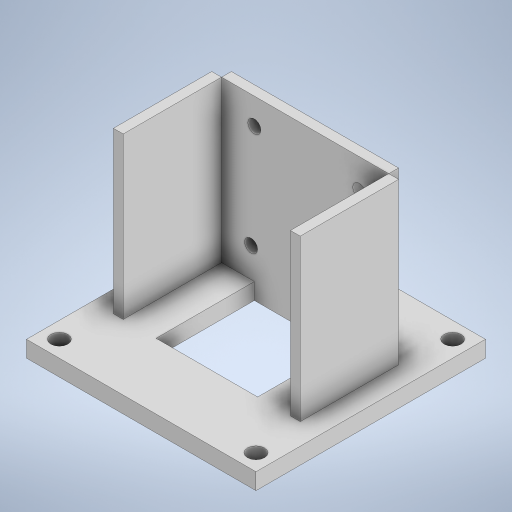
# Autodesk Inventor part: depth_camera_fastening
Saved by Autodesk Inventor 2024 (Build 280153000, 153)
## iProperties
Created: 2024-04-08
Part Number: depth_camera_fastening
Material: Genérico
Document SubType Name: Modeling
Designer: inigo
Density: 1 g/cm^3
Appearance: Valor por defecto
Author: inigo
Autodesk Inventor part; units mm, degrees
ref_plane "YZ Plane" through (0, 0, 0) normal (1, 0, 0) x (0, 1, 0)
ref_plane "XZ Plane" through (0, 0, 0) normal (0, 1, 0) x (-1, 0, 0)
ref_plane "XY Plane" through (0, 0, 0) normal (0, 0, 1) x (1, 0, 0)
sketch "Boceto1" plane through (0, 0, 0) normal (0, 1, 0) x (-1, 0, 0)
  line L0 (25.5, 15) -> (-25.5, 15)
  line L1 (-25.5, 15) -> (-25.5, -15)
  line L2 (-25.5, -15) -> (25.5, -15)
  line L3 (25.5, -15) -> (25.5, 15)
  line L4 (25.5, 15) -> (-25.5, -15) construction
  line L5 (-25.5, 15) -> (25.5, -15) construction
  line L6 (-15.5, 15) -> (-15.5, -15)
  line L7 (0, 15) -> (0, 11.847)
  line L8 (-25.5, 0) -> (-22.3332, 0)
  line L9 (25.5, 15) -> (25.5, -15)
  line L10 (15.5, 15) -> (15.5, -15)
  line L11 (25.5, 0) -> (22.3332, 0)
  line L12 (-25.5, -15) -> (-25.5, 15)
  line L13 (-25.5, 0) -> (-22.3332, 0)
  line L14 (-25.5, 15) -> (-25.5, -15)
  point P0 (0, 0)
  point P1 (31.5, 22.5)
  dimension "d2" = 10
  dimension "d21" = 51
  dimension "d22" = 30
  constraints: 30 end point, 5 symmetric about line, 4 midpoint, 2 horizontal, 2 parallel, 2 perpendicular, 2 point on line, 1 vertical
  measures "d2" distance between parallel lines of L6 L1
  measures "d21" distance between parallel lines of L3 L1
  measures "d22" distance between parallel lines of L0 L2
extrude "Extrusión1" add sketch "Boceto1" along normal blind 5 contours L3 L2 L10 L0 | L6 L2 L1 L0
sketch "Boceto4" plane through (0, 0, 0) normal (0, 1, 0) x (-1, 0, 0)
  line L0 (-28.5, 18) -> (28.5, 18)
  line L1 (28.5, 18) -> (28.5, -18)
  line L2 (28.5, -18) -> (-28.5, -18)
  line L3 (-28.5, -18) -> (-28.5, 18)
  line L4 (-28.5, 18) -> (28.5, -18) construction
  line L5 (28.5, 18) -> (-28.5, -18) construction
  line L6 (28.5, -15) -> (-28.5, -15)
  line L7 (-28.5, 15) -> (28.5, 15)
  line L8 (25.5, -18) -> (25.5, 18)
  line L9 (-25.5, 18) -> (-25.5, -18)
  line L10 (-25.5, -15) -> (-15.5, -15) projected
  point P0 (0, 0)
  point P1 (-25.5, -15)
  point P2 (-25.5, 15)
  point P3 (25.5, 15)
  point P4 (25.5, -15)
  dimension "d23" = 57
  dimension "d24" = 36
  dimension "d27" = 0
  constraints: 20 end point, 8 point on line, 5 perpendicular, 2 midpoint, 2 parallel, 1 horizontal
  measures "d23" distance of L1.end L2.end
  measures "d24" distance of L0.end L1.end
  measures "d27" distance between parallel lines of L6 L10
extrude "Extrusión4" add sketch "Boceto4" along normal blind 5 contours L0 L8 L7 L9 | L7 L9 L6 L3 | L7 L1 L6 L8 | L6 L8 L2 L9
sketch "Boceto5" plane through (0, 5, 0) normal (0, 1, 0) x (1, 0, 0)
  line L0 (25.5, 18) -> (-25.5, 18) projected
  line L1 (25.5, 15) -> (25.5, 18) projected
  line L2 (-25.5, 18) -> (25.5, 18)
  line L3 (25.5, 18) -> (25.5, 15)
  line L4 (25.5, 15) -> (-25.5, 15)
  line L5 (-25.5, 15) -> (-25.5, 18)
  point P0 (0, 0)
  constraints: 8 end point, 2 parallel, 1 horizontal, 1 perpendicular
extrude "Extrusión5" add sketch "Boceto5" along normal blind 49
sketch "Boceto6" plane through (-15.5, 0, -15) normal (0, 0, 1) x (1, 0, 0)
  circle A0 centre (32, 45) radius 2
  line L0 (41, 5) -> (41, 54) projected
  line L1 (-10, 54) -> (41, 54) projected
  line L2 (-10, 5) -> (-10, 54) projected
  line L3 (-10, 29.5) -> (15.5, 29.5)
  line L4 (15.5, 29.5) -> (15.5, 54)
  circle A1 centre (0, 46) radius 2
  circle A2 centre (-1, 14) radius 2
  circle A3 centre (31, 13) radius 2
  point P0 (15.5, 0)
  dimension "d30" = 4
  dimension "d31" = 9
  dimension "d32" = 9
  dimension "d35" = 360
  constraints: 4 centre point, 4 end point, 2 midpoint, 1 coincident, 1 horizontal, 9 other
  measures "d30" diameter of A0
  measures "d31" distance from line of L0 A0.centre
  measures "d32" distance from line of L1 A0.centre
extrude "Extrusión6" cut sketch "Boceto6" against normal blind 49 contours A0 | A1 | A2 | A3
sketch "Boceto7" plane through (0, 5, 0) normal (0, 1, 0) x (1, 0, 0)
  line L0 (-28.5, 15) -> (-28.5, -15) projected
  line L1 (-28.5, 15) -> (-25.5, 15)
  line L2 (-25.5, 15) -> (-25.5, -15)
  line L3 (-25.5, -15) -> (-28.5, -15)
  line L4 (-28.5, -15) -> (-28.5, 15)
  line L5 (28.5, 15) -> (25.5, 15) projected
  line L6 (25.5, -15) -> (28.5, -15) projected
  line L7 (28.5, 15) -> (25.5, 15)
  line L8 (25.5, 15) -> (25.5, -15)
  line L9 (25.5, -15) -> (28.5, -15)
  line L10 (28.5, -15) -> (28.5, 15)
  point P0 (0, 0)
  point P1 (25.5, -18)
  constraints: 16 end point, 4 parallel, 2 horizontal, 2 perpendicular
extrude "Extrusión7" add sketch "Boceto7" along normal blind 49
sketch "Boceto12" plane through (0, 0, 0) normal (0, -1, 0) x (1, 0, 0)
  line L0 (-35, -35) -> (35, -35)
  line L1 (35, -35) -> (35, 35)
  line L2 (35, 35) -> (-35, 35)
  line L3 (-35, 35) -> (-35, -35)
  line L4 (-35, -35) -> (35, 35) construction
  line L5 (35, -35) -> (-35, 35) construction
  line L6 (30, 30) -> (-30, 30)
  line L7 (-30, 30) -> (-30, -30)
  line L8 (-30, -30) -> (30, -30)
  line L9 (30, -30) -> (30, 30)
  line L10 (30, 30) -> (-30, -30) construction
  line L11 (-30, 30) -> (30, -30) construction
  circle A0 centre (-30, 30) radius 2.6
  circle A1 centre (30, 30) radius 2.6
  circle A2 centre (30, -30) radius 2.6
  circle A3 centre (-30, -30) radius 2.6
  line L12 (15.5, -15) -> (15.5, 15) projected
  line L13 (-15.5, -15) -> (15.5, -15)
  line L14 (15.5, -15) -> (15.5, 15)
  line L15 (15.5, 15) -> (-15.5, 15)
  line L16 (-15.5, 15) -> (-15.5, -15)
  line L17 (-15.5, -15) -> (15.5, 15) construction
  line L18 (15.5, -15) -> (-15.5, 15) construction
  point P0 (0, 0)
  point P1 (0, 0)
  dimension "d63" = 70
  dimension "d64" = 70
  dimension "d65" = 60
  dimension "d66" = 5.2
  dimension "d67" = 5.2
  dimension "d68" = 5.2
  dimension "d69" = 5.2
  constraints: 36 end point, 6 midpoint, 6 parallel, 4 centre point, 4 coincident, 3 horizontal, 3 perpendicular, 1 point on line
  measures "d63" distance of L2.end L2.start
  measures "d64" distance of L2.start L0.end
  measures "d65" distance of L7.end L6.end
  measures "d66" diameter of A0
  measures "d67" diameter of A1
  measures "d68" diameter of A2
  measures "d69" diameter of A3
extrude "Extrusión10" add sketch "Boceto12" against normal blind 5 contours L3 L2 L1 L0 | L6 A1 L9 A2 L8 A3 L7 A0
